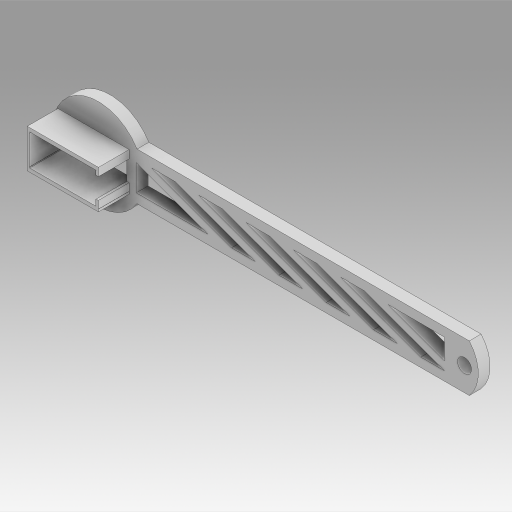
# Autodesk Inventor part: arm_v3-1_backup
Saved by Autodesk Inventor 2024.3 (Build 283343000, 343)
## iProperties
Created: 2024-07-19
Part Number: arm_v3-1_backup
Material: Ogólny
Document SubType Name: Modeling
Designer: User
Density: 1 g/cm^3
Appearance: Domyślna
Mass: 14.7779 g
Surface Area: 130.935 cm^2
Volume: 14.7779 cm^3
Author: User
Autodesk Inventor part; units mm, degrees
ref_plane "YZ Plane" through (0, 0, 0) normal (1, 0, 0) x (0, 1, 0)
ref_plane "XZ Plane" through (0, 0, 0) normal (0, 1, 0) x (-1, 0, 0)
ref_plane "XY Plane" through (0, 0, 0) normal (0, 0, 1) x (1, 0, 0)
sketch "Szkic1" plane through (0, 0, 0) normal (0, 1, 0) x (-1, 0, 0)
  line L0 (0, 0) -> (150, 0)
  line L1 (150, 0) -> (150, -5)
  line L2 (150, -5) -> (0, -5)
  line L3 (0, -5) -> (0, 0)
  dimension "d0" = 150
  dimension "d1" = 5
  constraints: 8 end point, 2 parallel, 1 horizontal, 1 perpendicular
  measures "d0" distance of L1.end L2.end
  measures "d1" distance of L0.end L1.end
extrude "Wyciągnięcie proste1" add sketch "Szkic1" along normal blind 20
sketch "Szkic2" plane through (0, 0, -5) normal (0, 0, -1) x (-1, 0, 0)
  line L0 (0, 0) -> (0, 20) projected
  circle A0 centre (0, 10) radius 2.95
  line L1 (0, 20) -> (-2, 20)
  line L2 (0, 0) -> (-2, 0)
  arc A1 (-2, 20) -> (-2, 0) centre (9.1803, 10) ccw
  line L3 (0, 10) -> (150, 10)
  line L4 (150, 10) -> (138.5, 10)
  line L5 (138.5, 10) -> (170.9, 10)
  line L6 (150, 0) -> (150, 20) projected
  line L7 (138.5, 10) -> (170.9, 10) construction
  line L8 (138.5, 10) -> (170.9, 10)
  line L9 (170.9, 10) -> (170.9, 16.16)
  line L10 (170.9, 16.16) -> (138.5, 16.16)
  line L11 (138.5, 16.16) -> (138.5, 10)
  line L12 (138.5, 10) -> (170.9, 10)
  line L13 (170.9, 10) -> (170.9, 3.84)
  line L14 (170.9, 3.84) -> (138.5, 3.84)
  line L15 (138.5, 3.84) -> (138.5, 10)
  line L16 (0, 0) -> (150, 0) projected
  line L17 (0, 20) -> (150, 20) projected
  arc A2 (138.5, 0) -> (138.5, 20) centre (154.9429, 10) ccw
  point P0 (150, 3.84)
  point P1 (150, 16.16)
  point P2 (0, 7.05)
  point P3 (0, 12.95)
  dimension "d4" = 5.9
  dimension "d5" = 2
  dimension "d6" = 2
  dimension "d7" = 15
  dimension "d8" = 150
  dimension "d9" = 11.5
  dimension "d10" = 32.4
  dimension "d11" = 0
  dimension "d12" = 6.16
  dimension "d13" = 6.16
  constraints: 28 end point, 6 horizontal, 4 parallel, 4 point on circle, 4 point on line, 3 centre point, 3 perpendicular, 1 collinear, 1 midpoint
  measures "d4" diameter of A0
  measures "d5" distance of L0.end L1.end
  measures "d6" distance of L0.start L2.end
  measures "d7" radius of A1
  measures "d8" distance of L3.start L3.end
  measures "d9" distance of L3.end L4.end
  measures "d10" distance of L4.end L5.end
  measures "d11" distance between parallel lines of L5 L7
  measures "d12" distance of L9.end L8.end
  measures "d13" distance of L12.end L13.end
extrude "Wyciągnięcie proste2" add sketch "Szkic2" against normal blind 5 contours L2 A1 L1 L0 A0 | L16 L6 L14 L13 L9 L10 L17 A2
sketch "Szkic3" plane through (2, 20, -5) normal (0, 0, -1) x (-1, 0, 0)
  arc A0 (2, -7.05) -> (2, -12.95) centre (2, -10) ccw projected
  circle A1 centre (2, -10) radius 2.95
  line L0 (152, -16.16) -> (152, -3.84) projected
  line L1 (152, -16.16) -> (150.5, -16.16)
  line L2 (150.5, -16.16) -> (150.5, -3.84)
  line L3 (150.5, -3.84) -> (152, -3.84)
  line L4 (140.5, -16.16) -> (10.5, -16.16)
  line L5 (10.5, -16.16) -> (10.5, -3.84)
  line L6 (10.5, -3.84) -> (140.5, -3.84)
  line L7 (140.5, -3.84) -> (140.5, -16.16)
  line L8 (150.5, -16.16) -> (150.3, -16.16)
  line L9 (150.3, -16.16) -> (150.3, -3.84)
  line L10 (150.3, -3.84) -> (150.5, -3.84)
  line L11 (152, -16.16) -> (140.5, -16.16)
  line L12 (140.5, -16.16) -> (140.5, -3.84)
  line L13 (140.5, -3.84) -> (152, -3.84)
  line L14 (152, -3.84) -> (152, -16.16)
  point P0 (2, -20)
  dimension "d16" = 1.5
  dimension "d17" = 130
  dimension "d18" = 12.32
  dimension "d21" = 0.2
  dimension "d24" = 11.5
  constraints: 28 end point, 5 perpendicular, 4 horizontal, 4 parallel, 1 centre point, 1 coincident, 1 vertical
  measures "d16" distance of L0.start L1.end
  measures "d17" distance of L5.end L6.end
  measures "d18" distance of L4.end L5.end
  measures "d21" distance of L1.end L8.end
  measures "d24" distance of L6.end L13.end
extrude "Wyciągnięcie proste3" cut sketch "Szkic3" against normal through all
sketch "Szkic5" plane through (2, 20, -5) normal (0, 0, -1) x (-1, 0, 0)
  circle A0 centre (2, -10) radius 2.95 projected
  line L0 (2, -10) -> (152, -10)
  line L1 (2, -10) -> (152, -10) construction
  circle A1 centre (152, -10) radius 5.0551
  line L2 (152, -10) -> (145.8, -10)
  line L3 (145.8, -10) -> (145.8, -3.84)
  line L4 (10.5, -3.84) -> (172.9, -3.84) projected
  line L5 (145.8, -3.84) -> (140.8, -3.84)
  line L6 (140.8, -3.84) -> (140.8, -16.16)
  line L7 (172.9, -16.16) -> (10.5, -16.16) projected
  line L8 (145.8, -10) -> (145.8, -16.16)
  line L9 (145.8, -16.16) -> (140.8, -16.16)
  line L10 (10.5, -16.16) -> (10.5, -3.84) projected
  line L11 (10.5, -16.16) -> (44.3489, -3.84)
  line L12 (10.5, -16.16) -> (46.5213, -16.16) construction
  line L13 (44.3489, -3.84) -> (54.3489, -3.84)
  line L14 (10.5, -16.16) -> (20.5, -16.16)
  line L15 (20.5, -16.16) -> (54.3489, -3.84)
  line L16 (20.5, -16.16) -> (30.5, -16.16)
  line L17 (54.3489, -3.84) -> (64.3489, -3.84)
  line L18 (64.3489, -3.84) -> (30.5, -16.16)
  line L19 (44.3489, -3.84) -> (34.3489, -3.84)
  line L20 (10.5, -16.16) -> (0.5, -16.16)
  line L21 (0.5, -16.16) -> (34.3489, -3.84)
  line L22 (40.5, -16.16) -> (74.3489, -3.84)
  line L23 (50.5, -16.16) -> (84.3489, -3.84)
  line L24 (94.3489, -3.84) -> (60.5, -16.16)
  line L25 (30.5, -16.16) -> (64.3489, -3.84)
  line L26 (70.5, -16.16) -> (104.3489, -3.84)
  line L27 (80.5, -16.16) -> (114.3489, -3.84)
  line L28 (124.3489, -3.84) -> (90.5, -16.16)
  line L29 (60.5, -16.16) -> (94.3489, -3.84)
  line L30 (100.5, -16.16) -> (134.3489, -3.84)
  line L31 (110.5, -16.16) -> (144.3489, -3.84)
  line L32 (90.5, -16.16) -> (124.3489, -3.84)
  point P0 (2, -20)
  point P1 (10.5, -12.5203)
  point P2 (60.5, -16.16)
  point P3 (140.8, -5.1317)
  dimension "d25" = 150
  dimension "d26" = 0
  dimension "d27" = 6.2
  dimension "d28" = 5
  dimension "d29" = 20
  dimension "d30" = 10
  dimension "d31" = 10
  dimension "d32" = 10
  dimension "d33" = 10
  dimension "d34" = 10
  dimension "d35" = 10
  dimension "d36" = 10
  dimension "d37" = 10
  dimension "d38" = 10
  dimension "d39" = 10
  dimension "d40" = 10
  dimension "d41" = 10
  dimension "d42" = 10
  dimension "d43" = 10
  dimension "d44" = 10
  dimension "d45" = 10
  dimension "d46" = 10
  dimension "d47" = 10
  dimension "d48" = 10
  dimension "d49" = 10
  dimension "d52" = 10
  dimension "d53" = 10
  constraints: 60 end point, 10 point on line, 4 horizontal, 2 equal length, 2 perpendicular, 2 vertical, 1 centre point, 1 coincident
  measures "d25" distance of L0.start L0.end
  measures "d26" distance between parallel lines of L0 L1
  measures "d27" distance of L2.start L2.end
  measures "d28" distance of L3.end L5.end
  measures "d29" angle of L12 L11
  measures "d30" distance of L11.end L13.end
  measures "d31" distance of L7.end L14.end
  measures "d32" distance of L14.end L16.end
  measures "d33" distance of L13.end L17.end
  measures "d34" distance of L11.end L19.end
  measures "d35" distance of L7.end L20.end
  measures "d36" distance of L22.end L23.end
  measures "d37" distance of L22.start L23.start
  measures "d38" distance of L23.start L24.end
  measures "d39" distance of L23.end L24.start
  measures "d40" distance of L22.end L25.end
  measures "d41" distance of L22.start L25.start
  measures "d42" distance of L26.end L27.end
  measures "d43" distance of L26.start L27.start
  measures "d44" distance of L27.start L28.end
  measures "d45" distance of L27.end L28.start
  measures "d46" distance of L26.end L29.end
  measures "d47" distance of L26.start L29.start
  measures "d48" distance of L30.end L31.end
  measures "d49" distance of L30.start L31.start
  measures "d52" distance of L30.end L32.end
  measures "d53" distance of L30.start L32.start
extrude "Wyciągnięcie proste4" add sketch "Szkic5" against normal blind 5 contours L21 L4 L11 L0 | L0 L11 L10 L21 | L15 L4 L18 L0 | L0 L18 L7 L15 | L22 L4 L23 L0 | L0 L23 L7 L22 | L24 L4 L26 L0 | L0 L26 L7 L24 | L27 L4 L28 L0 | L0 L28 L7 L27 | L30 L4 L6 L31 L0 | L0 L31 L7 L30 | L6 L31 L4 L3 L0 | L0 L8 L7 L6 | L6 L4 L31
sketch "Szkic6" plane through (-138.5, 0, 0) normal (0, 0, 1) x (1, 0, 0)
  line L0 (-32.4, 16.16) -> (-32.4, 3.84) projected
  line L1 (-5.3, 3.84) -> (-32.4, 3.84) projected
  line L2 (-32.4, 16.16) -> (-5.3, 16.16)
  line L3 (-5.3, 16.16) -> (-5.3, 3.84)
  line L4 (-5.3, 3.84) -> (-32.4, 3.84)
  line L5 (-32.4, 3.84) -> (-32.4, 16.16)
  line L6 (-32.4, 16.16) -> (-33.4, 16.16)
  line L7 (-33.4, 16.16) -> (-33.4, 17.16)
  line L8 (-5.3, 3.84) -> (-5.3, 2.84)
  line L9 (-5.3, 2.84) -> (-4.3, 2.84)
  line L10 (-33.4, 17.16) -> (-4.3, 17.16)
  line L11 (-4.3, 17.16) -> (-4.3, 2.84)
  line L12 (-4.3, 2.84) -> (-33.4, 2.84)
  line L13 (-33.4, 2.84) -> (-33.4, 17.16)
  point P0 (138.5, 0)
  point P1 (-33.4, 16.16)
  dimension "d56" = 1
  dimension "d57" = 1
  dimension "d58" = 1
  dimension "d59" = 1
  constraints: 24 end point, 4 parallel, 4 perpendicular, 3 horizontal, 1 vertical
  measures "d56" distance of L0.start L6.end
  measures "d57" distance of L6.end L7.end
  measures "d58" distance of L1.start L8.end
  measures "d59" distance of L8.end L9.end
extrude "Wyciągnięcie proste5" add sketch "Szkic6" along normal blind 13 contours L6 L7 L10 L11 L9 L8 L3 L2 | L0 L1 L8 L12 L13 L6
sketch "Szkic7" plane through (-142.8, 2.84, 0) normal (1, 0, 0) x (0, 0, -1)
  line L0 (-13, 0) -> (-13, 14.32) projected
  line L1 (0, 17.16) -> (0, -2.84) projected
  line L2 (-13, 11.9333) -> (0, 11.9333)
  line L3 (0, 11.9333) -> (0, 3.1608)
  line L4 (0, 3.1608) -> (-13, 3.1608)
  line L5 (-13, 3.1608) -> (-13, 11.9333)
  constraints: 8 end point, 2 parallel, 2 point on line, 1 horizontal, 1 perpendicular
extrude "Wyciągnięcie proste6" cut sketch "Szkic7" against normal blind 8.75
sketch "Szkic8" plane through (-138.5, 0, 0) normal (0, 0, 1) x (1, 0, 0)
  circle A0 centre (138.5, 10) radius 2.95 projected
  line L0 (138.5, 10) -> (-11.5, 10)
  circle A1 centre (-11.5, 10) radius 2.85
  line L1 (-14.35, 10) -> (-4.35, 10)
  line L2 (-4.35, 10) -> (-4.35, 16.6)
  line L3 (-4.35, 10) -> (2.25, 10) construction
  line L4 (-4.35, 10) -> (-4.35, 3.4)
  line L5 (-4.35, 16.6) -> (-32.35, 16.6)
  line L6 (-4.35, 16.6) -> (23.65, 16.6) construction
  line L7 (-32.35, 16.6) -> (-32.35, 3.4)
  line L8 (-32.35, 3.4) -> (-4.35, 3.4)
  point P0 (138.5, 0)
  dimension "d66" = 5.7
  dimension "d64" = 150
  dimension "d67" = 10
  dimension "d68" = 6.6
  dimension "d69" = 90
  dimension "d70" = 6.6
  dimension "d71" = 28
  dimension "d72" = 180
  dimension "d73" = 13.2
  constraints: 18 end point, 4 horizontal, 2 equal length, 2 vertical, 1 horizontal alignment, 1 perpendicular, 1 point on line, 2 other
  measures "d64" distance of L0.start L0.end
  measures "d67" distance of L1.start L1.end
  measures "d68" distance of L1.end L2.end
  measures "d69" angle of L3 L2
  measures "d70" distance of L1.end L4.end
  measures "d71" distance of L2.end L5.end
  measures "d72" angle of L5 L6
  measures "d73" distance of L5.end L7.end
extrude "Wyciągnięcie proste7" cut sketch "Szkic8" along normal blind 22.75 and the other way blind 20.75 contours L4 L8 L7 L5 L2
sketch "Szkic10" plane through (-138.5, 0, 0) normal (0, 0, 1) x (1, 0, 0)
  line L0 (-4.3, 17.16) -> (-4.3, 14.7733) projected
  line L1 (-4.3, 14.7733) -> (-3.3, 14.7733)
  line L2 (-3.3, 14.7733) -> (-3.3, 17.16)
  line L3 (-3.3, 17.16) -> (-4.3, 17.16)
  line L4 (-4.3, 17.16) -> (-4.3, 14.7733)
  line L5 (-4.35, 14.7733) -> (-4.35, 6.0008) projected
  line L6 (-4.35, 6.0008) -> (-3.35, 6.0008)
  line L7 (-3.35, 6.0008) -> (-3.35, 2.8422)
  line L8 (-3.35, 2.8422) -> (-4.35, 2.8422)
  line L9 (-4.35, 2.8422) -> (-4.35, 6.0008)
  line L10 (-33.4, 17.16) -> (-4.3, 17.16) projected
  line L11 (-33.4, 17.16) -> (-3.3, 17.16)
  line L12 (-3.3, 17.16) -> (-3.3, 18.16)
  line L13 (-3.3, 18.16) -> (-33.4, 18.16)
  line L14 (-33.4, 18.16) -> (-33.4, 17.16)
  line L15 (-33.4, 2.8422) -> (-3.3, 2.8422)
  line L16 (-3.3, 2.8422) -> (-3.3, 1.8422)
  line L17 (-3.3, 1.8422) -> (-33.4, 1.8422)
  line L18 (-33.4, 1.8422) -> (-33.4, 2.8422)
  point P0 (138.5, 0)
  point P1 (-3.3, 17.16)
  point P2 (-3.35, 2.8422)
  dimension "d78" = 1
  dimension "d79" = 1
  dimension "d80" = 1
  dimension "d81" = 1
  constraints: 32 end point, 8 parallel, 4 horizontal, 4 perpendicular, 3 point on line
  measures "d78" distance of L3.end L2.end
  measures "d79" distance of L7.end L8.end
  measures "d80" distance of L12.end L11.end
  measures "d81" distance of L15.end L16.end
extrude "Wyciągnięcie proste8" add sketch "Szkic10" along normal blind 13
sketch "Szkic11" plane through (2, 20, -5) normal (0, 0, -1) x (-1, 0, 0)
  circle A0 centre (2, -10) radius 2.95 projected
  line L0 (2, -10) -> (152, -10)
  line L1 (2, -10) -> (152, -10) construction
  circle A1 centre (152, -10) radius 2.4946
  point P0 (2, -20)
  dimension "d84" = 150
  dimension "d85" = 0
  constraints: 4 end point, 2 horizontal, 1 centre point, 1 coincident, 1 collinear
  measures "d84" distance of L0.start L0.end
  measures "d85" distance between parallel lines of L0 L1
